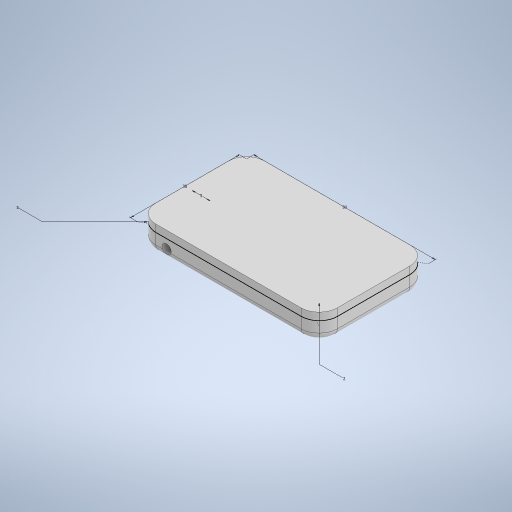
# Autodesk Inventor part: Base2
Saved by Autodesk Inventor 2024 (Build 280153000, 153)
## iProperties
Created: 2023-09-22
Part Number: Base2
Material: Genérico
Document SubType Name: Modeling
Designer: sergi
Density: 1 g/cm^3
Appearance: Valor por defecto
Author: sergi
Autodesk Inventor part; units mm, degrees
ref_plane "YZ Plane" through (0, 0, 0) normal (1, 0, 0) x (0, 1, 0)
ref_plane "XZ Plane" through (0, 0, 0) normal (0, 1, 0) x (-1, 0, 0)
ref_plane "XY Plane" through (0, 0, 0) normal (0, 0, 1) x (1, 0, 0)
sketch "Boceto1" plane through (0, 0, 0) normal (0, 1, 0) x (-1, 0, 0)
  line L0 (-20, 15) -> (20, 15)
  line L1 (25, 10) -> (25, -10)
  line L2 (20, -15) -> (-20, -15)
  line L3 (-25, -10) -> (-25, 10)
  line L4 (-25, 15) -> (25, -15) construction
  line L5 (25, 15) -> (-25, -15) construction
  line L6 (20, -10) -> (20, 10)
  line L7 (20, 10) -> (-18, 10)
  line L8 (-20, 8) -> (-20, -8)
  line L9 (-18, -10) -> (20, -10)
  arc A0 (25, 10) -> (20, 15) centre (20, 10) ccw
  arc A1 (20, -15) -> (25, -10) centre (20, -10) ccw
  arc A2 (-25, -10) -> (-20, -15) centre (-20, -10) ccw
  arc A3 (-20, 15) -> (-25, 10) centre (-20, 10) ccw
  arc A4 (-18, 10) -> (-20, 8) centre (-18, 8) ccw
  arc A5 (-20, -8) -> (-18, -10) centre (-18, -8) ccw
  point P0 (0, 0)
  dimension "d0" = 50
  dimension "d1" = 30
  dimension "d2" = 5
  dimension "d3" = 5
  dimension "d4" = 2
  constraints: 20 end point, 12 point on circle, 12 tangent, 8 point on line, 6 centre point, 4 equal radius, 4 parallel, 2 midpoint, 2 perpendicular, 1 horizontal, 3 other
  measures "d0" distance of L4.end L5.end
  measures "d1" distance of L5.start L4.end
  measures "d2" distance between parallel lines of L1 L6
  measures "d3" radius of A0
  measures "d4" radius of A4
extrude "Extrusión1" add sketch "Boceto1" along normal blind 2 contours L0 A0 L1 A1 L2 A2 L3 A3 | L9 A5 L8 A4 L7 L6
extrude "Extrusión2" add sketch "Boceto1" against normal blind 5
sketch "Boceto3" plane through (20, 2, -15) normal (0, 0, -1) x (-1, 0, 0)
  line L0 (2, -2) -> (40, -2) projected
  line L1 (2, -2) -> (2, -7) projected
  line L2 (40, -7) -> (2, -7) projected
  line L3 (40, -2) -> (40, -7) projected
  line L4 (40, -4.5) -> (37, -4.5)
  circle A0 centre (37, -4.5) radius 2.5
  circle A1 centre (37, -4.5) radius 1.25
  point P0 (20, -2)
  dimension "d9" = 3
  dimension "d10" = 2.5
  constraints: 2 centre point, 2 coincident, 2 end point, 1 midpoint, 1 parallel, 1 tangent
  measures "d9" distance of L4.start L4.end
  measures "d10" diameter of A1
extrude "Extrusión3" cut sketch "Boceto3" against normal through all contours A1
fillet "Empalme1" radius 2 8 edges at (-23.5355, -5, -13.5355) (0, -5, -15) (23.5355, -5, -13.5355) (25, -5, 0) (23.5355, -5, 13.5355) (0, -5, 15) (-23.5355, -5, 13.5355) (-25, -5, 0)
